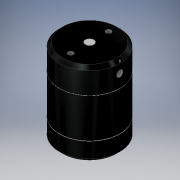
# Autodesk Inventor part: Motor
Saved by Autodesk Inventor 2019.4 (Build 234330000, 330)
## iProperties
Created: 2019-10-15
Part Number: Motor
Material: Generic
Document SubType Name: Modeling
Designer: Jorian Bruslind
Density: 1 g/cm^3
Appearance: Default
Author: Jorian Bruslind
Autodesk Inventor part; units mm, degrees
sketch "Sketch1" plane through (0, 0, 0) normal (0, 1, 0) x (-1, 0, 0)
  circle A0 centre (0, 0) radius 14
  dimension "d0" = 28
  constraints: 1 centre point, 1 coincident
  measures "d0" diameter of A0
extrude "Extrusion1" add sketch "Sketch1" along normal blind 38.4
chamfer "Chamfer1" distance 1.5 angle 45 2 edges at (14, 38.4, 0) (14, 0, 0)
sketch "Sketch2" plane through (0, 38.4, 0) normal (0, 1, 0) x (1, 0, 0)
  circle A0 centre (0, 0) radius 2
  dimension "d6" = 4
  constraints: 1 centre point, 1 coincident
  measures "d6" diameter of A0
extrude "Extrusion2" add sketch "Sketch2" along normal blind 0.1
sketch "Sketch3" plane through (0, 38.4, 0) normal (0, 1, 0) x (1, 0, 0)
  line L0 (0, 0) -> (0, 8.75)
  circle A0 centre (0, 8.75) radius 1.25
  line L1 (0, 0) -> (0, -8.75)
  line L2 (0, 0) -> (8.75, 0) construction
  circle A1 centre (0, -8.75) radius 1.25
  dimension "d9" = 8.75
  dimension "d10" = 2.5
  dimension "d11" = 8.75
  dimension "d12" = 90
  dimension "d13" = 2.5
  constraints: 6 end point, 2 centre point, 2 coincident, 2 vertical, 1 horizontal, 1 perpendicular
  measures "d9" distance of L0.start L0.end
  measures "d10" diameter of A0
  measures "d11" distance of L0.start L1.end
  measures "d12" angle of L1 L2
  measures "d13" diameter of A1
extrude "Extrusion4" cut sketch "Sketch3" against normal blind 5
thread "Thread1" size "M2.5x0.45" class "6H" standard "ANSI Metric M Profile" full length
thread "Thread2" size "M2.5x0.45" class "6H" standard "ANSI Metric M Profile" full length
ref_plane "Work Plane1" through (0, 36.9, 0) normal (0, 1, 0) x (1, 0, 0)
sketch "Sketch6" plane through (0, 36.9, 0) normal (0, 1, 0) x (1, 0, 0)
  line L0 (0.125, 13.75) -> (-0.125, 13.75)
  line L1 (-0.125, 13.75) -> (-0.125, 14.25)
  line L2 (-0.125, 14.25) -> (0.125, 14.25)
  line L3 (0.125, 14.25) -> (0.125, 13.75)
  circle A0 centre (0, 0) radius 14 projected
  line L4 (0.125, 13.75) -> (-0.125, 14.25) construction
  line L5 (-0.125, 13.75) -> (0.125, 14.25) construction
  point P0 (0, 14)
  dimension "d25" = 0.25
  dimension "d26" = 0.5
  constraints: 12 end point, 2 midpoint, 2 parallel, 1 horizontal, 1 perpendicular, 1 vertical alignment, 1 other
  measures "d25" distance of L1.end L2.end
  measures "d26" distance of L0.end L1.end
extrude "Extrusion5" add sketch "Sketch6" against normal blind 1 contours L0 L1 A0 L3 | A0 L1 L2 L3 picked at (-0.0139, 13.8333)
ref_plane "Work Plane2" through (-0.125, 0, -13.9994) normal (-0.0089, 0, -1) x (-1, 0, 0.0089)
sketch "Sketch7" plane through (-0.125, 0, -13.9994) normal (-0.0089, 0, -1) x (-1, 0, 0.0089)
  line L0 (0, 36.9) -> (0, 26.9)
  line L1 (0, 36.9) -> (0, 35.9) projected
  line L2 (0, 36.9) -> (10, 36.9) construction
  line L3 (-87.9645, 27) -> (87.9645, 27)
  line L4 (87.9645, 27) -> (87.9645, 26.8)
  line L5 (87.9645, 26.8) -> (-87.9645, 26.8)
  line L6 (-87.9645, 26.8) -> (-87.9645, 27)
  line L7 (-87.9645, 27) -> (87.9645, 26.8) construction
  line L8 (87.9645, 27) -> (-87.9645, 26.8) construction
  line L9 (0, 26.8) -> (0, 8.8)
  line L10 (0, 26.8) -> (18, 26.8) construction
  line L11 (0, 8.8) -> (0, 8.675)
  line L12 (0, 8.8) -> (0.125, 8.8) construction
  line L13 (-87.9645, 8.55) -> (87.9645, 8.55)
  line L14 (87.9645, 8.55) -> (87.9645, 8.8)
  line L15 (87.9645, 8.8) -> (-87.9645, 8.8)
  line L16 (-87.9645, 8.8) -> (-87.9645, 8.55)
  line L17 (-87.9645, 8.55) -> (87.9645, 8.8) construction
  line L18 (87.9645, 8.55) -> (-87.9645, 8.8) construction
  point P0 (0, 0)
  dimension "d29" = 10
  dimension "d30" = 90
  dimension "d31" = 175.929
  dimension "d32" = 0.2
  dimension "d33" = 18
  dimension "d34" = 90
  dimension "d35" = 0.125
  dimension "d36" = 90
  dimension "d37" = 175.929
  dimension "d38" = 0.25
  constraints: 36 end point, 5 horizontal, 5 midpoint, 5 perpendicular, 4 parallel, 2 vertical, 1 collinear
  measures "d29" distance of L0.start L0.end
  measures "d30" angle of L0 L2
  measures "d31" distance of L4.end L5.end
  measures "d32" distance of L3.end L4.end
  measures "d33" distance of L9.start L9.end
  measures "d34" angle of L9 L10
  measures "d35" distance of L9.end L11.end
  measures "d36" angle of L11 L12
  measures "d37" distance of L15.end L14.end
  measures "d38" distance of L14.end L13.end
sketch3d "3D Sketch1"
extrude "Extrusion6" cut sketch "Sketch7" against normal blind 28
sketch "Sketch8" plane through (0, 38.4, 0) normal (0, 1, 0) x (1, 0, 0)
  line L0 (0, 0) -> (14, 0)
  line L1 (14.125, 0.125) -> (13.875, 0.125)
  line L2 (13.875, 0.125) -> (13.875, -0.125)
  line L3 (13.875, -0.125) -> (14.125, -0.125)
  line L4 (14.125, -0.125) -> (14.125, 0.125)
  line L5 (14.125, 0.125) -> (13.875, -0.125) construction
  line L6 (13.875, 0.125) -> (14.125, -0.125) construction
  dimension "d41" = 14
  dimension "d42" = 0.25
  dimension "d43" = 0.25
  constraints: 14 end point, 2 horizontal, 2 midpoint, 2 parallel, 1 perpendicular
  measures "d41" distance of L0.start L0.end
  measures "d42" distance of L3.end L2.end
  measures "d43" distance of L2.end L1.end
extrude "Extrusion7" add sketch "Sketch8" against normal blind 1
ref_plane "Work Plane3" through (14, 0, 0) normal (1, 0, 0) x (0, 1, 0)
sketch "Sketch9" plane through (14, 0, 0) normal (1, 0, 0) x (0, 1, 0)
  line L0 (38.4, 0.125) -> (38.4, -0.125) projected
  line L1 (38.4, -0.125) -> (38.4, 0)
  line L2 (38.4, 0) -> (32.9, 0)
  line L3 (38.4, 0) -> (43.9, 0) construction
  circle A0 centre (32.9, 0) radius 1.5
  point P0 (0, 0)
  dimension "d46" = 5.5
  dimension "d47" = 180
  dimension "d48" = 3
  constraints: 6 end point, 1 centre point, 1 coincident, 1 collinear, 1 horizontal, 1 midpoint, 1 perpendicular
  measures "d46" distance of L1.end L2.end
  measures "d47" angle of L2 L3
  measures "d48" diameter of A0
extrude "Extrusion8" cut sketch "Sketch9" against normal blind 5
thread "Thread3" size "M3x0.5" class "6H" standard "ANSI Metric M Profile" full length
pattern_circular "Circular Pattern1" count 2 over 360 about axis through (0, 0, 0) along (0, 1, 0) of "Extrusion8"
thread "Thread4" size "M3x0.5" class "6H" standard "ANSI Metric M Profile" full length
sketch "Sketch10" plane through (0, 0, 0) normal (0, -1, 0) x (1, 0, 0)
  line L0 (0, 0) -> (5, 0)
  line L1 (13.9194, -1.5) -> (9, -1.5) projected
  line L2 (0, 0) -> (5, 0) construction
  line L3 (5, 0) -> (5, 5)
  line L4 (5, 0) -> (10, 0) construction
  circle A0 centre (5, 5) radius 1.25
  circle A1 centre (5, -5) radius 1.25
  circle A2 centre (-5, 5) radius 1.25
  circle A3 centre (-5, -5) radius 1.25
  dimension "d58" = 5
  dimension "d59" = 0
  dimension "d60" = 5
  dimension "d61" = 90
  dimension "d62" = 2.5
  dimension "d65" = 10
  dimension "d68" = 10
  constraints: 8 end point, 4 centre point, 3 horizontal, 2 equal length, 2 vertical, 1 coincident, 1 parallel, 6 other
  measures "d58" distance of L0.start L0.end
  measures "d59" distance between parallel lines of L0 L2
  measures "d60" distance of L2.end L3.end
  measures "d61" angle of L4 L3
  measures "d62" diameter of A0
  measures "d65" distance of A0.centre A1.centre
  measures "d68" distance of A0.centre A2.centre
extrude "Extrusion9" cut sketch "Sketch10" against normal blind 5
thread "Thread5" size "M2.5x0.45" class "6H" standard "ANSI Metric M Profile" full length
thread "Thread6" size "M2.5x0.45" class "6H" standard "ANSI Metric M Profile" full length
thread "Thread7" size "M2.5x0.45" class "6H" standard "ANSI Metric M Profile" full length
thread "Thread8" size "M2.5x0.45" class "6H" standard "ANSI Metric M Profile" full length
sketch "Sketch11" plane through (0, 0, 0) normal (0, -1, 0) x (1, 0, 0)
  line L0 (0, 0) -> (0, -7)
  line L1 (0, 0) -> (7, 0) construction
  line L2 (-5, -14) -> (5, -14)
  line L3 (-3, -7) -> (-3, -9)
  line L4 (-3, -7) -> (-1, -7) construction
  line L5 (-3, -9) -> (-5, -9) construction
  line L6 (-3, -9) -> (-3, -7) construction
  line L7 (-3, -9) -> (-5, -9)
  line L8 (3, -9) -> (3, -7)
  line L9 (3, -9) -> (5, -9)
  arc A0 (-3, -7) -> (-5, -9) centre (-3, -9) ccw
  arc A1 (5, -9) -> (3, -7) centre (3, -9) ccw
  line L10 (-3, -7) -> (3, -7)
  line L11 (-5, -9) -> (-5, -14)
  line L12 (5, -9) -> (5, -14)
  dimension "d81" = 7
  dimension "d82" = 90
  dimension "d87" = 2
  dimension "d88" = 90
  dimension "d89" = 90
  dimension "d90" = 6
  dimension "d91" = 5
  dimension "d92" = 10
  dimension "d93" = 7
  constraints: 26 end point, 4 point on circle, 3 coincident, 3 horizontal, 3 perpendicular, 3 symmetric about line, 2 centre point, 2 equal length, 2 vertical
  measures "d81" distance of L0.start L0.end
  measures "d82" angle of L0 L1
  measures "d87" distance of L3.start L3.end
  measures "d88" angle of L3 L4
  measures "d89" angle of L6 L5
  measures "d90" distance of L3.start L8.end
  measures "d91" distance of L5.end L2.start
  measures "d92" distance of L2.start L2.end
  measures "d93" distance between parallel lines of L1 L10
extrude "Extrusion10" cut sketch "Sketch11" against normal blind 5.25
sketch "Sketch12" plane through (0, 5.25, 0) normal (0, -1, 0) x (1, 0, 0)
  line L0 (-3, -7) -> (3, -7) projected
  line L1 (0, -7) -> (0, -9)
  line L2 (0, -9) -> (0, -11.5)
  line L3 (0.125, -14.25) -> (0.125, -13.9994) projected
  line L4 (0, -9) -> (2.5, -9) construction
  line L5 (1.25, -13.25) -> (-1.25, -13.25)
  line L6 (-1.25, -13.25) -> (-1.25, -9.75)
  line L7 (-1.25, -9.75) -> (1.25, -9.75)
  line L8 (1.25, -9.75) -> (1.25, -13.25)
  line L9 (1.25, -13.25) -> (-1.25, -9.75) construction
  line L10 (-1.25, -13.25) -> (1.25, -9.75) construction
  line L11 (0, -11.5) -> (-3, -11.5)
  line L12 (-1.75, -13.25) -> (-4.25, -13.25)
  line L13 (-4.25, -13.25) -> (-4.25, -9.75)
  line L14 (-4.25, -9.75) -> (-1.75, -9.75)
  line L15 (-1.75, -9.75) -> (-1.75, -13.25)
  line L16 (-1.75, -13.25) -> (-4.25, -9.75) construction
  line L17 (-4.25, -13.25) -> (-1.75, -9.75) construction
  line L18 (0, -11.5) -> (3, -11.5)
  line L19 (4.25, -13.25) -> (1.75, -13.25)
  line L20 (1.75, -13.25) -> (1.75, -9.75)
  line L21 (1.75, -9.75) -> (4.25, -9.75)
  line L22 (4.25, -9.75) -> (4.25, -13.25)
  line L23 (4.25, -13.25) -> (1.75, -9.75) construction
  line L24 (1.75, -13.25) -> (4.25, -9.75) construction
  point P0 (0, 0)
  dimension "d96" = 2
  dimension "d97" = 2.5
  dimension "d98" = 90
  dimension "d99" = 2.5
  dimension "d100" = 3.5
  dimension "d101" = 3
  dimension "d102" = 2.5
  dimension "d103" = 3.5
  dimension "d104" = 3
  dimension "d105" = 2.5
  dimension "d106" = 3.5
  constraints: 46 end point, 7 midpoint, 7 parallel, 6 horizontal, 4 perpendicular, 1 vertical
  measures "d96" distance of L1.start L1.end
  measures "d97" distance of L1.end L2.end
  measures "d98" angle of L2 L4
  measures "d99" distance of L6.end L7.end
  measures "d100" distance of L5.end L6.end
  measures "d101" distance of L2.end L11.end
  measures "d102" distance of L13.end L14.end
  measures "d103" distance of L12.end L13.end
  measures "d104" distance of L2.end L18.end
  measures "d105" distance of L20.end L21.end
  measures "d106" distance of L19.end L20.end
extrude "Extrusion11" add sketch "Sketch12" along normal blind 0.1
body "Solid1"
